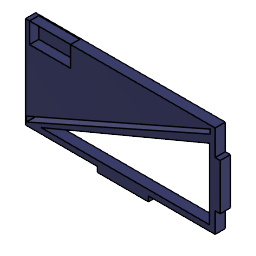
side_wall (Autodesk Fusion 360 design; units mm, degrees)
part number: 2026-06-29-20-59-02-690
Autodesk Fusion 360 part; units mm, degrees
derive "DerivedContext1"
sketch "Sketch1" plane through (0, 0, 0) normal (0, 1, 0) x (1, 0, 0)
  line L0 (0, -95.0301) -> (190, -95.0301)
  line L1 (190, -95.0301) -> (190, -0.0301)
  line L2 (190, -0.0301) -> (0, -0.0301)
  line L3 (0, -0.0301) -> (0, -95.0301)
  line L4 (190, -0.0301) -> (120, -0.0301)
  line L5 (120, -0.0301) -> (120, -5.0301)
  line L6 (120, -5.0301) -> (190, -5.0301)
  line L7 (190, -5.0301) -> (190, -0.0301)
  line L8 (0, 0) -> (70, 0)
  line L9 (70, 0) -> (70, -5)
  line L10 (70, -5) -> (0, -5)
  line L11 (0, -5) -> (0, 0)
  line L12 (190, -95.0301) -> (185, -95.0301)
  line L13 (185, -95.0301) -> (185, -70.0301)
  line L14 (185, -70.0301) -> (190, -70.0301)
  line L15 (190, -70.0301) -> (190, -95.0301)
  line L16 (190, -0.0301) -> (185, -0.0301)
  line L17 (185, -0.0301) -> (185, -25.0301)
  line L18 (185, -25.0301) -> (190, -25.0301)
  line L19 (190, -25.0301) -> (190, -0.0301)
  dimension "d1" = 95
  dimension "d2" = 190
  dimension "d7" = 5
  dimension "d8" = 70
  dimension "d9" = 70
  dimension "d10" = 50
  dimension "d11" = 25
  dimension "d12" = 5
  dimension "d13" = 45
  constraint horizontal L0
  constraint vertical L1
  constraint horizontal L2
  constraint vertical L3
  constraint horizontal L4
  constraint vertical L5
  constraint horizontal L6
  constraint vertical L7
  constraint horizontal L8
  constraint vertical L9
  constraint horizontal L10
  constraint vertical L11
  constraint coincident L8.start L11.end
  constraint equal L5 L9
  constraint horizontal L12
  constraint vertical L13
  constraint horizontal L14
  constraint vertical L15
  constraint horizontal L16
  constraint vertical L17
  constraint horizontal L18
  constraint vertical L19
  constraint equal L14 L18
  measures "d1" distance of L0.start L2.end
  measures "d2" distance of L1.end L2.end
  measures "d7" distance of L4 L6
  measures "d8" distance of L9 L11
  measures "d9" distance of L1.end L4.end
  measures "d10" distance of L5 L9
  measures "d11" distance of L16.end L17.end
  measures "d12" distance of L17.end L18.end
  measures "d13" distance of L14 L18
extrude "Extrude3" add sketch "Sketch1" along normal blind 10 contours L0 L1 L2 L3 L5 L6 L9 L10 L13 L14 L17 L18
sketch "Sketch3" plane through (0, 0, 0) normal (0, 1, 0) x (1, 0, 0)
  line L0 (0.9177, -13.0377) -> (0.9177, -8.0377)
  line L1 (0.9177, -8.0377) -> (180.1295, -87.4047)
  line L2 (180.1295, -87.4047) -> (180.1295, -91.6563)
  line L3 (180.1295, -91.6563) -> (0.9177, -13.0377)
  point P0 (185, -95.0301)
  dimension "d42" = 5
  dimension "d43" = 5
  dimension "d59" = 196
  constraint vertical L0
  measures "d42" distance of L1 P0
  measures "d43" distance of L0.start L0.end
  measures "d59" distance of L0.end L1.end
extrude "Extrude5" cut sketch "Sketch3" along normal through all
sketch "Sketch4" plane through (0, 0, 0) normal (0, 1, 0) x (1, 0, 0)
  line L0 (4, -94.9905) -> (44, -94.9905)
  line L1 (44, -94.9905) -> (44, -74.9905)
  line L2 (44, -74.9905) -> (4, -74.9905)
  line L3 (4, -74.9905) -> (4, -94.9905)
  line L4 (0, -0.0301) -> (0, -95.0301)
  dimension "d46" = 20
  dimension "d47" = 40
  dimension "d48" = 4
  constraint horizontal L0
  constraint vertical L1
  constraint horizontal L2
  constraint vertical L3
  measures "d46" distance of L0.end L1.end
  measures "d47" distance of L1.end L2.end
  measures "d48" distance of L3 L4
extrude "Extrude6" cut sketch "Sketch4" along normal blind 9
sketch "Sketch6" plane through (0, 0, 0) normal (0, 1, 0) x (1, 0, 0)
  line L0 (179.5, -79.3384) -> (15.2575, -10.5)
  line L1 (15.2575, -10.5) -> (179.5, -10.5)
  line L2 (179.5, -10.5) -> (179.5, -79.3384)
  line L3 (70, -5) -> (0, -5)
  line L4 (185, -95.0301) -> (185, -70.0301)
  dimension "d56" = 5.5
  dimension "d57" = 5.5
  constraint horizontal L1
  constraint perpendicular L1 L2
  measures "d56" distance of L1 L3
  measures "d57" distance of L2 L4
extrude "Extrude8" cut sketch "Sketch6" along normal through all
